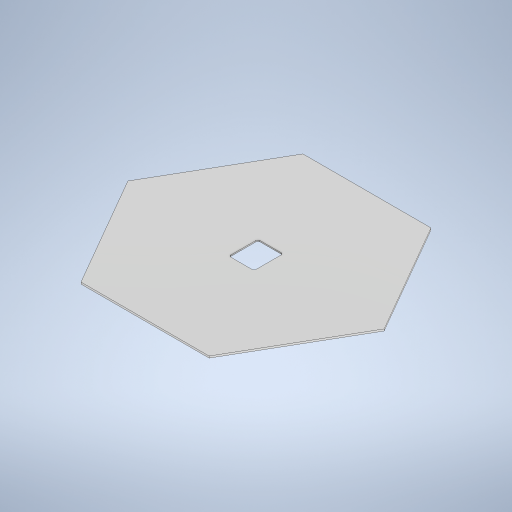
# Autodesk Inventor part: AEON.AcrylicTop
Saved by Autodesk Inventor 2023.2 (Build 272271000, 271)
## iProperties
Created: 2022-07-15
Part Number: AEON.AcrylicTop
Material: Generic
Document SubType Name: Modeling
Designer: delh
Mass: 320.759 g
Surface Area: 2366.97 cm^2
Volume: 320.759 cm^3
Density: 1 g/cm^3
Appearance: Default
Author: delh
Autodesk Inventor part; units mm, degrees
ref_plane "YZ Plane" through (0, 0, 0) normal (1, 0, 0) x (0, 1, 0)
ref_plane "XZ Plane" through (0, 0, 0) normal (0, 1, 0) x (-1, 0, 0)
ref_plane "XY Plane" through (0, 0, 0) normal (0, 0, 1) x (1, 0, 0)
sketch "Sketch1" plane through (0, 0, 0) normal (0, 0, 1) x (1, 0, 0)
  line L0 (213.0422, 0) -> (106.5211, -184.5)
  line L1 (106.5211, -184.5) -> (-106.5211, -184.5)
  line L2 (-106.5211, -184.5) -> (-213.0422, 0)
  line L3 (-213.0422, 0) -> (-106.5211, 184.5)
  line L4 (-106.5211, 184.5) -> (106.5211, 184.5)
  line L5 (106.5211, 184.5) -> (213.0422, 0)
  point P0 (0, 0)
  point P1 (0, 0)
  dimension "d0" = 369
  constraints: 12 end point, 1 coincident, 13 other
  measures "d0" distance between parallel lines of L1 L4
extrude "Extrusion1" add sketch "Sketch1" along normal blind 3
sketch "Sketch3" plane through (0, 0, 3) normal (0, 0, 1) x (1, 0, 0)
  line L0 (20.9, -20.75) -> (20.9, 20.75) projected
  arc A0 (17.5, -24.15) -> (20.9, -20.75) centre (17.5, -20.75) ccw projected
  line L1 (-17.5, -24.15) -> (17.5, -24.15) projected
  arc A1 (-20.9, -20.75) -> (-17.5, -24.15) centre (-17.5, -20.75) ccw projected
  line L2 (-20.9, 20.75) -> (-20.9, -20.75) projected
  arc A2 (-17.5, 24.15) -> (-20.9, 20.75) centre (-17.5, 20.75) ccw projected
  line L3 (17.5, 24.15) -> (-17.5, 24.15) projected
  arc A3 (20.9, 20.75) -> (17.5, 24.15) centre (17.5, 20.75) ccw projected
  line L4 (213.6196, 0) -> (106.8098, -185) projected
  line L5 (106.8098, 185) -> (213.6196, 0) projected
  line L6 (-106.8098, 185) -> (106.8098, 185) projected
  line L7 (-213.6196, 0) -> (-106.8098, 185) projected
  line L8 (-106.8098, -185) -> (-213.6196, 0) projected
  line L9 (106.8098, -185) -> (-106.8098, -185) projected
  point P0 (0, 0)
extrude "Extrusion2" cut sketch "Sketch3" against normal blind 3 contours A0 L1 A1 L2 A2 L3 A3 L0
sketch "Sketch4" plane through (0, 0, 0) normal (0, 0, -1) x (-1, 0, 0)
  line L0 (49.5995, 87.1474) -> (49.5995, -46.8) projected
  line L1 (48.3995, -48) -> (-73.3995, -48) projected
  line L2 (-74.5995, -46.8) -> (-74.5995, 87.1474) projected
  arc A0 (-39.8967, 142.8769) -> (-74.5995, 87.1474) centre (-12.5, 87.1474) ccw projected
  arc A1 (49.5995, 87.1474) -> (14.8967, 142.8769) centre (-12.5, 87.1474) ccw projected
  line L3 (-82.5, -56) -> (57.5, -56)
  line L4 (57.5, -56) -> (57.5, 151)
  line L5 (57.5, 151) -> (-82.5, 151)
  line L6 (-82.5, 151) -> (-82.5, -56)
  line L7 (-39.8967, 142.8769) -> (14.8967, 142.8769)
  point P0 (0, 0)
  dimension "d5" = 140
  dimension "d6" = 207
  dimension "d8" = 57.5
  dimension "d11" = 56
  constraints: 10 end point, 2 horizontal, 2 parallel, 1 perpendicular
  measures "d5" distance between parallel lines of L4 L6
  measures "d6" distance between parallel lines of L5 L3
  measures "d8" distance from line of L4 point (0, 0)
  measures "d11" distance from line of L3 point (0, 0)
extrude "Extrusion3" cut sketch "Sketch4" against normal blind 1
body "Solid1"
